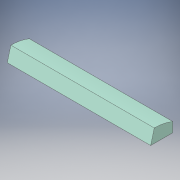
# Autodesk Inventor part: spacebar-keycap_mockup_cherrymx
Saved by Autodesk Inventor 2016 (Build 200138000, 138)
## iProperties
Created: 2016-12-10
Part Number: spacebar-keycap_mockup_cherrymx
Material: Generic
Document SubType Name: Modeling
Designer: Cemra JC
Density: 1 g/cm^3
Appearance: Default
Author: Cemra JC
Autodesk Inventor part; units mm, degrees
ref_plane "YZ Plane" through (0, 0, 0) normal (1, 0, 0) x (0, 1, 0)
ref_plane "XZ Plane" through (0, 0, 0) normal (0, 1, 0) x (-1, 0, 0)
ref_plane "XY Plane" through (0, 0, 0) normal (0, 0, 1) x (1, 0, 0)
sketch "Spacebar base" plane through (0, 0, 0) normal (0, 1, 0) x (-1, 0, 0)
  line L0 (58.825, 9.05) -> (-58.825, 9.05)
  line L1 (-58.825, 9.05) -> (-58.825, -9.05)
  line L2 (-58.825, -9.05) -> (58.825, -9.05)
  line L3 (58.825, -9.05) -> (58.825, 9.05)
  line L4 (58.825, 9.05) -> (-58.825, -9.05) construction
  line L5 (-58.825, 9.05) -> (58.825, -9.05) construction
  point P0 (0, 0)
  dimension "d0" = 117.65
  dimension "d1" = 18.1
  constraints: 12 end point, 2 midpoint, 2 parallel, 1 horizontal, 1 perpendicular
  measures "d0" distance of L2.end L1.end
  measures "d1" distance of L1.end L0.end
extrude "Spacebar Bulk" add sketch "Spacebar base" along normal blind 11
sketch "Curve Profile" plane through (58.825, 0, 9.05) normal (1, 0, 0) x (0, 0, -1)
  line L0 (0, 0) -> (18.1, 0) projected
  line L1 (0, 0) -> (2.9474, 11)
  line L2 (0, 11) -> (18.1, 11) projected
  line L3 (18.1, 0) -> (18.1, 11) projected
  arc A0 (18.1, 8) -> (2.9474, 11) centre (2.9474, -28.7667) ccw
  line L4 (0, 0) -> (0, 11) projected
  line L5 (18.1, 8) -> (18.1, 0)
  line L6 (18.1, 0) -> (0, 0)
  point P0 (9.05, 0)
  dimension "d4" = 15
  dimension "d9" = 8
  constraints: 6 end point, 2 collinear, 2 point on circle, 2 point on line, 1 centre point, 1 tangent
  measures "d4" angle of L1 L4
  measures "d9" distance of L0.end L5.start
extrude "Curve Cutaway" cut sketch "Curve Profile" against normal up to surface (117.65 mm away) contours L1 A0 L3 L0 keep common part
shell "Inner Shell" thickness 1.5 removed faces 1 at (19.6083, 0, 3.0167)
ref_plane "PoleBase Plane" through (57.325, 9.4828, 4.9562) normal (0, 0.9995512, -0.0299579) x (-1, 0, 0)
sketch "Center Circle" plane through (57.325, 9.4828, 4.9562) normal (0, 0.9995512, -0.0299579) x (-1, 0, 0)
  circle A0 centre (57.325, -5.238) radius 2.77
  dimension "d11" = 5.54
  constraints: 1 centre point, 1 coincident
  measures "d11" diameter of A0
extrude "Pole Extrusion" add sketch "Center Circle" against normal up to surface surface through (0, 0, 0) normal (0, 1, 0)
sketch "Sketch4" plane through (0, 0, 0) normal (0, -1, 0) x (1, 0, 0)
  line L0 (-2.2, 0.675) -> (2.2, 0.675)
  line L1 (2.2, 0.675) -> (2.2, -0.675)
  line L2 (2.2, -0.675) -> (-2.2, -0.675)
  line L3 (-2.2, -0.675) -> (-2.2, 0.675)
  line L4 (-2.2, 0.675) -> (2.2, -0.675) construction
  line L5 (2.2, 0.675) -> (-2.2, -0.675) construction
  line L6 (0.675, 2.2) -> (-0.675, 2.2)
  line L7 (-0.675, 2.2) -> (-0.675, -2.2)
  line L8 (-0.675, -2.2) -> (0.675, -2.2)
  line L9 (0.675, -2.2) -> (0.675, 2.2)
  line L10 (0.675, 2.2) -> (-0.675, -2.2) construction
  line L11 (-0.675, 2.2) -> (0.675, -2.2) construction
  point P0 (0, 0)
  dimension "d14" = 4.4
  dimension "d15" = 1.35
  dimension "d16" = 1.35
  dimension "d17" = 4.4
  constraints: 24 end point, 4 midpoint, 4 parallel, 2 horizontal, 2 perpendicular
  measures "d14" distance of L1.end L2.end
  measures "d15" distance of L0.end L1.end
  measures "d16" distance of L8.end L7.end
  measures "d17" distance of L7.end L6.end
extrude "Extrusion4" cut sketch "Sketch4" against normal blind 5
equation "\"d0\" = b_space"
equation "\"d1\" = k_width"
equation "\"d10\" = k_wthick"
equation "\"d11\" = k_poledia"
equation "\"d14\" = k_cmxl"
equation "\"d15\" = k_cmxw"
equation "\"d16\" = k_cmxw"
equation "\"d17\" = k_cmxl"
equation "\"k_width\" = 18.1"
equation "\"k_height\" = 18"
equation "\"k_height_t\" = 16"
equation "\"k_taper1\" = 1.5"
equation "\"k_taper2\" = 0.5"
equation "\"k_staper\" = 1"
equation "\"k_sradius\" = 4"
equation "\"k_ltaper\" = 1.5"
equation "\"k_lradius\" = 6"
equation "\"k_radius\" = 6"
equation "\"k_wthick\" = 1.5"
equation "\"k_ribthick\" = 1.5"
equation "\"k_ribheight\" = 5"
equation "\"k_poleoff\" = 2.2625"
equation "\"k_poledia\" = 5.54"
equation "\"k_cmxw\" = 1.35"
equation "\"k_cmxl\" = 4.4"
equation "\"s_bwidth\" = 15.6"
equation "\"s_poleh\" = 3.6"
equation "\"s_polebw\" = 5.5"
equation "\"s_polebl\" = 7"
equation "\"b_pad\" = 1"
equation "\"b_tab\" = 27.15"
equation "\"b_caps\" = 31.675"
equation "\"b_lshift\" = 40.725"
equation "\"b_rshift\" = 49.775"
equation "\"b_ctrl\" = 22.625"
equation "\"b_space\" = 117.65"
equation "\"b_width\" = 286.5"
equation "\"b_height\" = 77.4"
body "Solid1"
